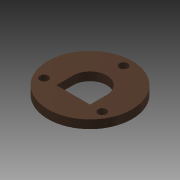
# Autodesk Inventor part: 刀夹片
Saved by Autodesk Inventor 2015 (Build 190159000, 159)
## iProperties
Created: 2017-05-18
Part Number: 刀夹片
Material: 常规
Document SubType Name: Modeling
Designer: Administrator
Density: 1 g/cm^3
Appearance: 青铜 - 缎光
Author: Administrator
Autodesk Inventor part; units mm, degrees
ref_plane "YZ Plane" through (0, 0, 0) normal (1, 0, 0) x (0, 1, 0)
ref_plane "XZ Plane" through (0, 0, 0) normal (0, 1, 0) x (-1, 0, 0)
ref_plane "XY Plane" through (0, 0, 0) normal (0, 0, 1) x (1, 0, 0)
sketch "草图1" plane through (0, 0, 0) normal (0, 0, 1) x (1, 0, 0)
  circle A0 centre (0, 0) radius 25
  dimension "d0" = 50
  constraints: 1 centre point, 1 coincident
  measures "d0" diameter of A0
extrude "拉伸1" add sketch "草图1" along normal blind 5
sketch "草图2" plane through (0, 0, 5) normal (0, 0, 1) x (1, 0, 0)
  circle A0 centre (0, 0) radius 10
  line L0 (-10, 0) -> (-10, -10)
  line L1 (-10, -10) -> (10, -10)
  line L2 (10, -10) -> (10, 0)
  dimension "d3" = 20
  constraints: 6 end point, 3 tangent, 2 perpendicular, 2 point on circle, 1 centre point, 1 coincident, 1 vertical
  measures "d3" diameter of A0
extrude "拉伸2" cut sketch "草图2" against normal through all
sketch "草图3" plane through (0, 0, 5) normal (0, 0, 1) x (1, 0, 0)
  circle A0 centre (-17.3205, -10) radius 2.5
  circle A1 centre (17.3205, -10) radius 2.5
  circle A2 centre (0, 20) radius 2.5
  line L0 (0, 0) -> (0, 20)
  line L1 (0, 0) -> (-17.3205, -10)
  line L2 (0, 0) -> (17.3205, -10)
  dimension "d6" = 5
  dimension "d7" = 5
  dimension "d8" = 5
  dimension "d9" = 20
  dimension "d10" = 120
  dimension "d11" = 120
  constraints: 6 end point, 3 centre point, 2 equal length, 1 vertical
  measures "d6" diameter of A0
  measures "d7" diameter of A1
  measures "d8" diameter of A2
  measures "d9" distance of L0.start L0.end
  measures "d10" angle of L2 L0
  measures "d11" angle of L2 L1
extrude "拉伸3" cut sketch "草图3" against normal through all
